Autodesk Fusion 360 part; units mm, degrees
note: some values were not read from the file. Set by a fixed rule: which face or edge a step refers to.
(part 2 of 5)
sketch "Sketch11" plane through (-60, 0, 0) normal (-1, 0, 0) x (0, 0, 1)
  line L0 (-42, 0) -> (42, 0)
  line L1 (42, 31) -> (-42, 31)
  line L2 (-42, 7) -> (-42, 10)
  line L3 (-42, 8.5) -> (41.5, 8.5) construction
  circle A0 centre (-29.5, 8.5) radius 1.5
  circle A1 centre (-24.5, 8.5) radius 1.5
  circle A2 centre (-19.5, 8.5) radius 1.5
  circle A3 centre (-14.5, 8.5) radius 1.5
  circle A4 centre (29.5, 8.5) radius 1.5
  circle A5 centre (24.5, 8.5) radius 1.5
  circle A6 centre (19.5, 8.5) radius 1.5
  circle A7 centre (14.5, 8.5) radius 1.5
  circle A8 centre (-29.5, 13.5) radius 1.5
  circle A9 centre (-24.5, 13.5) radius 1.5
  circle A10 centre (-19.5, 13.5) radius 1.5
  circle A11 centre (-14.5, 13.5) radius 1.5
  circle A12 centre (-29.5, 18.5) radius 1.5
  circle A13 centre (-24.5, 18.5) radius 1.5
  circle A14 centre (-19.5, 18.5) radius 1.5
  circle A15 centre (-14.5, 18.5) radius 1.5
  circle A16 centre (29.5, 13.5) radius 1.5
  circle A17 centre (24.5, 13.5) radius 1.5
  circle A18 centre (19.5, 13.5) radius 1.5
  circle A19 centre (14.5, 13.5) radius 1.5
  circle A20 centre (29.5, 18.5) radius 1.5
  circle A21 centre (24.5, 18.5) radius 1.5
  circle A22 centre (19.5, 18.5) radius 1.5
  circle A23 centre (14.5, 18.5) radius 1.5
  line L4 (-6, 5) -> (-6, 16)
  line L5 (-6, 16) -> (10, 16)
  line L6 (10, 16) -> (10, 5)
  line L7 (10, 5) -> (-6, 5)
  line L8 (42, 0) -> (42, 31)
  line L9 (-42, 31) -> (-42, 0)
  dimension "d84" = 3
  dimension "d87" = 15
  dimension "d88" = 10
  dimension "d91" = -15
  dimension "d92" = 10
  constraint midpoint L2 L3.start
  constraint coincident L3 A0.centre
  constraint coincident L3 A4.centre
  constraint equal A0 A4
  measures "d84" diameter of A0
extrude "Extrude10" cut sketch "Sketch11" against normal up to surface (8 mm away) contours A0 | A1 | A2 | A3 | A4 | A5 | A6 | A7 | A8 | A9 | A10 | A11 | A12 | A13 | A14 | A15 | A16 | A17 | A18 | A19 | A20 | A21 | A22 | A23 bodies 1
fillet "Fillet1" [suppressed]
fillet "Fillet2" [suppressed]
equation "d3 = d1 / 2"
equation "d4 = d2 / 2"
equation "d8 = d7"
equation "d9 = d7"
equation "d10 = d7"
equation "d18 = d17"
equation "d19 = d17"
equation "d20 = d17"
equation "d21 = d17 + 4 mm"
equation "d22 = d21"
equation "d23 = d21"
equation "d24 = d21"
equation "d25 = 8.00 mm"
equation "d27 = d25 - 1 mm"
equation "d32 = 2 mm"
equation "d33 = d32"
equation "d34 = d25"
equation "d40 = d39"
equation "d41 = d39"
equation "d42 = d39"
equation "d62 = d60 / 2"
equation "d63 = d61 / 2"
equation "d66 = d64"
equation "d68 = d67"
equation "d69 = d67"
equation "d70 = d67"

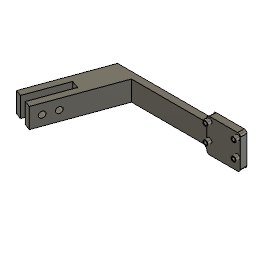
design "Camera Arm"
Autodesk Fusion 360 part; units mm, degrees
sketch "Sketch1" plane through (0, 0, 0) normal (0, 0, 1) x (1, 0, 0)
  circle A0 centre (10.5, -3.138) radius 1.2
  line L0 (-10.5, 12.5) -> (10.5, 12.5)
  arc A1 (-12.5, -10.5) -> (-10.5, -12.5) centre (-10.5, -10.5) ccw
  circle A2 centre (-10.5, -3.138) radius 1.2
  arc A3 (10.5, -12.5) -> (12.5, -10.5) centre (10.5, -10.5) ccw
  circle A4 centre (-10.5, 9.362) radius 1.2
  arc A5 (-10.5, 12.5) -> (-12.5, 10.5) centre (-10.5, 10.5) ccw
  line L1 (-12.5, -10.5) -> (-12.5, 10.5)
  line L2 (12.5, 10.5) -> (12.5, -10.5)
  arc A6 (12.5, 10.5) -> (10.5, 12.5) centre (10.5, 10.5) ccw
  circle A7 centre (10.5, 9.362) radius 1.2
  line L3 (10.5, -12.5) -> (-10.5, -12.5)
  point P0 (-12.5, 12.5)
  point P1 (12.5, 12.5)
  point P2 (-12.5, -12.5)
  dimension "d1" = 25
  dimension "d2" = 25
  dimension "d3" = 2.4
  dimension "d4" = 2
  dimension "d5" = 2
  dimension "d6" = 2
  dimension "d7" = 2
  dimension "d8" = 2
  dimension "d9" = 2
  dimension "d10" = 2
  dimension "d11" = 12.5
  dimension "d12" = 12.5
  dimension "d13" = 21.862
  dimension "d14" = 21.862
  dimension "d15" = 9.362
  dimension "d16" = 9.362
  dimension "d17" = 12.5
  dimension "d18" = 12.5
  constraint horizontal L0
  constraint vertical L2
  constraint horizontal L3
  constraint vertical L1
  constraint equal A2 A4
  constraint equal A0 A2
  constraint equal A0 A7
  constraint coincident P0 L0
  constraint coincident P0 L1
  constraint tangent L0 A5
  constraint tangent A5 L1
  constraint coincident P1 L0
  constraint coincident P1 L2
  constraint tangent L0 A6
  constraint tangent L2 A6
  constraint equal A5 A6
  constraint coincident P2 L3
  constraint coincident P2 L1
  constraint tangent A1 L3
  constraint tangent A1 L1
  constraint tangent A3 L2
  constraint tangent A3 L3
  measures "d1" distance of P0 P1
  measures "d2" distance of P0 P2
  measures "d3" diameter of A4
  measures "d4" distance of A7.centre L2
  measures "d5" distance of A0.centre L2
  measures "d6" distance of A2.centre L1
  measures "d7" distance of A4.centre L1
  measures "d8" radius of A5
  measures "d9" radius of A1
  measures "d10" radius of A3
  measures "d11" distance of origin L1
  measures "d12" distance of origin L0
  measures "d13" distance of A7.centre L3
  measures "d14" distance of A4.centre L3
  measures "d15" distance of A0.centre L3
  measures "d16" distance of A2.centre L3
  measures "d17" distance of origin L1
  measures "d18" distance of origin L0
extrude "Extrude1" add sketch "Sketch1" along normal blind 5
sketch "Sketch2" plane through (0, 0, 5) normal (0, 0, 1) x (1, 0, 0)
  circle A0 centre (-10.5, 9.362) radius 1.2
  circle A1 centre (10.5, -3.138) radius 1.2
  circle A2 centre (-10.5, -3.138) radius 1.2
  circle A3 centre (10.5, 9.362) radius 1.2
  arc A4 (12.5, 10.5) -> (10.5, 12.5) centre (10.5, 10.5) ccw
  line L0 (10.5, 12.5) -> (-10.5, 12.5)
  arc A5 (-10.5, 12.5) -> (-12.5, 10.5) centre (-10.5, 10.5) ccw
  line L1 (-12.5, 10.5) -> (-12.5, -10.5)
  arc A6 (-12.5, -10.5) -> (-10.5, -12.5) centre (-10.5, -10.5) ccw
  line L2 (-10.5, -12.5) -> (10.5, -12.5)
  arc A7 (10.5, -12.5) -> (12.5, -10.5) centre (10.5, -10.5) ccw
  line L3 (12.5, -10.5) -> (12.5, 10.5)
  circle A8 centre (-10.5, 9.362) radius 1.85
  circle A9 centre (10.5, 9.362) radius 1.85
  circle A10 centre (10.5, -3.138) radius 1.85
  circle A11 centre (-10.5, -3.138) radius 1.85
  dimension "d21" = 3.7
  dimension "d22" = 3.7
  dimension "d23" = 3.7
  dimension "d24" = 3.7
  constraint concentric A0 A8
  constraint concentric A3 A9
  constraint concentric A1 A10
  constraint concentric A2 A11
  measures "d21" diameter of A8
  measures "d22" diameter of A9
  measures "d23" diameter of A10
  measures "d24" diameter of A11
extrude "Extrude2" add sketch "Sketch2" along normal blind 3 contours A8 | A9 | A10 | A11
sketch "Sketch3" plane through (-12.5, 0, 0) normal (-1, 0, 0) x (0, 0, 1)
  line L0 (0, 10.5) -> (0, -10.5)
  line L1 (0, -10.5) -> (5, -10.5)
  line L2 (5, -10.5) -> (5, 10.5)
  line L3 (5, 10.5) -> (0, 10.5)
  line L4 (0, 7.5) -> (5, 7.5)
  line L5 (5, 7.5) -> (5, -7.5)
  line L6 (5, -7.5) -> (0, -7.5)
  line L7 (0, -7.5) -> (0, 7.5)
  dimension "d29" = 3
  dimension "d30" = 3
  constraint horizontal L4
  constraint vertical L5
  constraint horizontal L6
  constraint vertical L7
  constraint coincident L2 L5.end
  constraint coincident L0 L4.start
  measures "d29" distance of L3 L4
  measures "d30" distance of L1 L6
extrude "Extrude3" add sketch "Sketch3" along normal blind 68 contours L0 L2 L4 L5 L6 L7
fillet "Fillet1" radius 3 2 edges at (-12.5, 7.5, 2.5) (-12.5, -7.5, 2.5)
sketch "Sketch5" plane through (0, 7.5, 0) normal (0, 1, 0) x (-1, 0, 0)
  line L0 (15.5, 5) -> (15.5, 0)
  line L1 (15.5, 0) -> (80.5, 0)
  line L2 (80.5, 0) -> (80.5, 5)
  line L3 (80.5, 5) -> (15.5, 5)
  line L4 (80.5, 0) -> (94.2374, 0)
  line L5 (94.2374, 0) -> (80.5, 5)
  line L6 (84.001, 0) -> (85.1985, 3.2899)
  dimension "d38" = 20
  dimension "d39" = 5
  dimension "d40" = 5
  constraint coincident L1.end L2.start
  constraint perpendicular L2 L4
  constraint coincident L2.end L3.start
  constraint coincident L4 L6.start
  constraint coincident L5 L6.end
  constraint perpendicular L5 L6
  measures "d38" angle of L4 L5
  measures "d39" distance of L1.end L2.end
  measures "d40" distance of L2.end L6.end
extrude "Extrude5" add sketch "Sketch5" against normal up to surface (15 mm away) contours L2 L4 L5 L6
sketch "Sketch6" plane through (-11.0237, 0, 30.2873) normal (-0.34202, 0, 0.939693) x (0.939693, 0, 0.34202)
  line L0 (-78.9352, -7.5) -> (-73.9352, -7.5)
  line L1 (-73.9352, -7.5) -> (-73.9352, 7.5)
  line L2 (-73.9352, 7.5) -> (-78.9352, 7.5)
  line L3 (-78.9352, 7.5) -> (-78.9352, -7.5)
  line L4 (-78.9352, 7.5) -> (-73.9352, 7.5)
  line L5 (-73.9352, 7.5) -> (-73.9352, -7.5)
  line L6 (-73.9352, -7.5) -> (-78.9352, -7.5)
  line L7 (-78.9352, -7.5) -> (-78.9352, 7.5)
  constraint horizontal L4
  constraint vertical L5
  constraint horizontal L6
  constraint vertical L7
  constraint coincident L0.end L1.start
  constraint coincident L2.end L3.start
extrude "Extrude6" add sketch "Sketch6" along normal blind 55.398
sketch "Sketch7" plane through (-69.4763, 0, -25.2873) normal (0.939693, 0, 0.34202) x (0.34202, 0, -0.939693)
  line L0 (-32.2311, -7.5) -> (-32.2311, 7.5)
  line L1 (-32.2311, 7.5) -> (-87.6291, 7.5)
  line L2 (-87.6291, 7.5) -> (-87.6291, -7.5)
  line L3 (-87.6291, -7.5) -> (-32.2311, -7.5)
  line L4 (-87.6291, 0) -> (-32.2311, 0) construction
  circle A0 centre (-80.1291, 0) radius 2.25
  circle A1 centre (-70.1291, 0) radius 2.25
  dimension "d45" = 4.5
  dimension "d46" = 4.5
  dimension "d47" = 7.5
  dimension "d48" = 10
  constraint midpoint L2 L4.start
  constraint midpoint L0 L4.end
  constraint coincident L4 A0.centre
  constraint coincident L4 A1.centre
  measures "d45" diameter of A0
  measures "d46" diameter of A1
  measures "d47" distance of L2 A0.centre
  measures "d48" distance of A0.centre A1.centre
extrude "Extrude7" cut sketch "Sketch7" against normal up to surface (5 mm away) contours A0 | A1
sketch "Sketch8" plane through (0, 7.5, 0) normal (0, 1, 0) x (-1, 0, 0)
  line L0 (15.5, 5) -> (15.5, 0)
  line L1 (15.5, 0) -> (84.001, 0)
  line L2 (84.001, 0) -> (104.1457, 55.347)
  line L3 (104.1457, 55.347) -> (99.4472, 57.0571)
  line L4 (99.4472, 57.0571) -> (80.5, 5)
  line L5 (80.5, 5) -> (15.5, 5)
  line L6 (74.0085, 5) -> (93.7151, 59.1434)
  line L7 (93.7151, 59.1434) -> (89.0166, 60.8535)
  line L8 (89.0166, 60.8535) -> (68.6876, 5)
  line L9 (99.4472, 57.0571) -> (93.7151, 59.1434) construction
  dimension "d51" = 6.1
  dimension "d52" = 5
  constraint coincident L5 L6.start
  constraint perpendicular L6 L7
  constraint coincident L5 L8.end
  constraint parallel L4 L6
  constraint perpendicular L7 L8
  constraint coincident L3.end L4.start
  constraint perpendicular L4 L9
  measures "d51" distance of L4 L6
  measures "d52" distance of L6.end L7.end
extrude "Extrude8" add sketch "Sketch8" against normal up to surface (15 mm away) contours L5 L6 L7 L8
sketch "Sketch9" plane through (-59.0457, 0, -21.4909) normal (0.939693, 0, 0.34202) x (0.34202, 0, -0.939693)
  line L0 (-87.6291, -7.5) -> (-28.191, -7.5)
  line L1 (-28.191, -7.5) -> (-28.191, 7.5)
  line L2 (-28.191, 7.5) -> (-87.6291, 7.5)
  line L3 (-87.6291, 7.5) -> (-87.6291, -7.5)
  circle A0 centre (-80.1291, 0) radius 2.25
  circle A1 centre (-70.1291, 0) radius 2.25
extrude "Extrude9" cut sketch "Sketch9" against normal up to surface (5 mm away) contours A0 | A1
sketch "Sketch10" plane through (0, 7.5, 0) normal (0, 1, 0) x (-1, 0, 0)
  line L0 (15.5, 5) -> (15.5, 0)
  line L1 (15.5, 0) -> (84.001, 0)
  line L2 (84.001, 0) -> (104.1457, 55.347)
  line L3 (104.1457, 55.347) -> (99.4472, 57.0571)
  line L4 (99.4472, 57.0571) -> (80.5, 5)
  line L5 (80.5, 5) -> (74.0085, 5)
  line L6 (74.0085, 5) -> (93.7151, 59.1434)
  line L7 (93.7151, 59.1434) -> (89.0166, 60.8535)
  line L8 (89.0166, 60.8535) -> (68.6876, 5)
  line L9 (68.6876, 5) -> (15.5, 5)
  line L10 (89.0505, 28.4923) -> (83.3184, 30.5786)
  dimension "d57" = 30.398
  constraint coincident L4 L10.start
  constraint coincident L6 L10.end
  constraint perpendicular L6 L10
  measures "d57" distance of L3 L10
extrude "Extrude10" add sketch "Sketch10" against normal up to surface (15 mm away) contours L4 L5 L6 L10
equation "d17 = d11"
equation "d18 = d12"
equation "d22 = d21"
equation "d23 = d21"
equation "d24 = d21"
equation "d30 = d29"
equation "d40 = d39"
equation "d43 = 19.898 mm + 7.5 mm + 28 mm"
equation "d46 = d45"
equation "d57 = d43 - 25 mm"

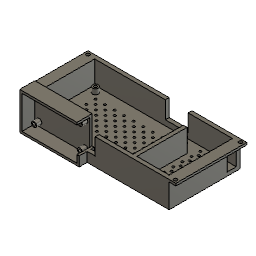
design "PCB Case"
Autodesk Fusion 360 part; units mm, degrees
sketch "Sketch1" plane through (0, 0, 0) normal (0, 1, 0) x (1, 0, 0)
  line L0 (-72.5, 44.98) -> (120.5, 44.98)
  line L1 (120.5, 44.98) -> (120.5, -49.32)
  line L2 (120.5, -49.32) -> (-72.5, -49.32)
  line L3 (-72.5, -49.32) -> (-72.5, 44.98)
  line L4 (-67.5, 39.83) -> (67.5, 39.83)
  line L5 (67.5, 39.83) -> (67.5, -39.83)
  line L6 (67.5, -39.83) -> (-67.5, -39.83)
  line L7 (-67.5, -39.83) -> (-67.5, 39.83)
  circle A0 centre (-58.42, 31.75) radius 1.9
  circle A1 centre (-58.42, -31.75) radius 1.9
  circle A2 centre (58.42, 31.75) radius 1.9
  circle A3 centre (58.42, -31.75) radius 1.9
  circle A4 centre (-58.42, 31.75) radius 3.9
  circle A5 centre (58.42, 31.75) radius 3.9
  circle A6 centre (58.42, -31.75) radius 3.9
  circle A7 centre (-58.42, -31.75) radius 3.9
  line L8 (72.5, 39.83) -> (115.5, 39.83)
  line L9 (115.5, 39.83) -> (115.5, -44.17)
  line L10 (115.5, -44.17) -> (72.5, -44.17)
  line L11 (72.5, -44.17) -> (72.5, 39.83)
  line L12 (67.5, 39.83) -> (72.5, 39.83) construction
  dimension "d1" = 135
  dimension "d2" = 67.5
  dimension "d3" = 79.66
  dimension "d4" = 39.83
  dimension "d5" = 5.15
  dimension "d8" = 5
  dimension "d9" = 58.42
  dimension "d10" = 58.42
  dimension "d11" = 58.42
  dimension "d12" = 58.42
  dimension "d13" = 31.75
  dimension "d14" = 31.75
  dimension "d15" = 31.75
  dimension "d16" = 31.75
  dimension "d17" = 3.8
  dimension "d18" = 3.8
  dimension "d19" = 3.8
  dimension "d20" = 3.8
  dimension "d21" = 7.8
  dimension "d22" = 7.8
  dimension "d23" = 7.8
  dimension "d24" = 7.8
  dimension "d111" = 43
  dimension "d112" = 84
  dimension "d113" = 5.15
  dimension "d114" = 5
  dimension "d115" = 5
  constraint horizontal L0
  constraint vertical L1
  constraint horizontal L2
  constraint vertical L3
  constraint horizontal L4
  constraint vertical L5
  constraint horizontal L6
  constraint vertical L7
  constraint concentric A0 A4
  constraint concentric A2 A5
  constraint concentric A3 A6
  constraint concentric A1 A7
  constraint horizontal L8
  constraint vertical L9
  constraint horizontal L10
  constraint vertical L11
  constraint horizontal L12
  measures "d1" distance of L4.start L4.end
  measures "d2" distance of origin L5
  measures "d3" distance of L4.start L6.end
  measures "d4" distance of origin L4
  measures "d5" distance of L0 L4
  measures "d8" distance of L3 L7
  measures "d9" horizontal distance of origin A0.centre
  measures "d10" horizontal distance of origin A2.centre
  measures "d11" horizontal distance of origin A1.centre
  measures "d12" horizontal distance of origin A3.centre
  measures "d13" vertical distance of origin A0.centre
  measures "d14" vertical distance of origin A2.centre
  measures "d15" vertical distance of origin A1.centre
  measures "d16" vertical distance of origin A3.centre
  measures "d17" diameter of A0
  measures "d18" diameter of A2
  measures "d19" diameter of A1
  measures "d20" diameter of A3
  measures "d21" diameter of A4
  measures "d22" diameter of A5
  measures "d23" diameter of A7
  measures "d24" diameter of A6
  measures "d111" distance of L8.start L8.end
  measures "d112" distance of L8.end L9.end
  measures "d113" distance of L2 L10
  measures "d114" distance of L1 L9
  measures "d115" distance of L5 L11
extrude "Extrude1" add sketch "Sketch1" along normal blind 5 contours L4 L5 L6 L7 | A4 | A5 | A6 | A7 | L8 L9 L10 L11 makes body 1 at (-18.887, 0, 10.2448) makes body 2 at (86.8333, 0, 16.17)
extrude "Extrude3" add sketch "Sketch1" along normal blind 35 contours L0 L1 L2 L3 bodies 1 2
extrude "Extrude15" add sketch "Sketch1" along normal blind 5 contours A0 | A1 | A2 | A3 bodies 1
extrude "Extrude16" add sketch "Sketch1" along normal blind 12 contours A4 | A5 | A6 | A7 bodies 1
sketch "Sketch11" plane through (0, 35, 0) normal (0, 1, 0) x (-1, 0, 0)
  line L0 (-67.5, 39.83) -> (67.5, 39.83)
  line L1 (67.5, 39.83) -> (67.5, -39.83)
  line L2 (67.5, -39.83) -> (-67.5, -39.83)
  line L3 (-67.5, -39.83) -> (-67.5, 39.83)
  line L4 (-115.5, 44.17) -> (-72.5, 44.17)
  line L5 (-72.5, 44.17) -> (-72.5, -39.83)
  line L6 (-72.5, -39.83) -> (-115.5, -39.83)
  line L7 (-115.5, -39.83) -> (-115.5, 44.17)
  line L8 (72.5, 49.32) -> (-120.5, 49.32)
  line L9 (-120.5, 49.32) -> (-120.5, -44.98)
  line L10 (-120.5, -44.98) -> (72.5, -44.98)
  line L11 (72.5, -44.98) -> (72.5, 49.32)
  line L12 (72.5, 49.32) -> (-67.5, 49.32)
  line L13 (-67.5, 49.32) -> (-67.5, 44.83)
  line L14 (-67.5, 44.83) -> (72.5, 44.83)
  line L15 (72.5, 44.83) -> (72.5, 49.32)
  line L16 (-67.5, 44.83) -> (-67.5, 39.83)
  dimension "d117" = 5
  constraint horizontal L12
  constraint vertical L13
  constraint horizontal L14
  constraint vertical L15
  constraint coincident L8.start L11.end
  constraint coincident L0.start L3.end
  constraint vertical L16
  measures "d117" distance of L0 L14
extrude "Extrude11" cut sketch "Sketch11" against normal up to surface (35 mm away) contours L8 L11 L12 L13 L14 L15 bodies 1
sketch "Sketch2" plane through (0, 35, 0) normal (0, 1, 0) x (-1, 0, 0)
  line L0 (-67.5, 39.83) -> (67.5, 39.83)
  line L1 (67.5, 39.83) -> (67.5, -39.83)
  line L2 (67.5, -39.83) -> (-67.5, -39.83)
  line L3 (-67.5, -39.83) -> (-67.5, 39.83)
  line L4 (-67.5, 49.32) -> (-120.5, 49.32)
  line L5 (-120.5, 49.32) -> (-120.5, -44.98)
  line L6 (-120.5, -44.98) -> (72.5, -44.98)
  line L7 (72.5, -44.98) -> (72.5, 44.83)
  line L8 (81.5, -44.98) -> (-129.5, -44.98)
  line L9 (-129.5, -44.98) -> (-129.5, 49.32)
  line L10 (81.5, 44.83) -> (81.5, -44.98)
  circle A0 centre (77, 40.33) radius 2.25
  circle A1 centre (77, -40.48) radius 2.25
  circle A2 centre (-125, -40.98) radius 2.25
  circle A3 centre (-125, 45.32) radius 2.25
  line L11 (-115.5, 44.17) -> (-72.5, 44.17)
  line L12 (-72.5, 44.17) -> (-72.5, -39.83)
  line L13 (-72.5, -39.83) -> (-115.5, -39.83)
  line L14 (-115.5, -39.83) -> (-115.5, 44.17)
  line L15 (-67.5, 44.83) -> (-67.5, 49.32)
  line L16 (72.5, 44.83) -> (-67.5, 44.83)
  line L17 (-129.5, 49.32) -> (-120.5, 49.32)
  line L18 (72.5, 44.83) -> (81.5, 44.83)
  point P0 (-24, -44.98)
  dimension "d33" = 9
  dimension "d39" = 4.5
  dimension "d40" = 4.5
  dimension "d41" = 4.5
  dimension "d42" = 4.5
  dimension "d43" = 4
  dimension "d44" = 4.5
  dimension "d46" = 4.5
  dimension "d47" = 4.5
  dimension "d48" = 4.5
  dimension "d50" = 4.5
  dimension "d116" = 9
  dimension "d121" = 4
  dimension "d122" = 4.5
  constraint horizontal L8
  constraint vertical L9
  constraint vertical L10
  constraint midpoint L6 P0
  constraint coincident L8 P0
  constraint coincident L4.end L5.start
  constraint perpendicular L5 L17
  constraint coincident L7.end L16.start
  constraint horizontal L18
  measures "d33" distance of L7 L10
  measures "d39" distance of L10 A1.centre
  measures "d40" distance of L8 A1.centre
  measures "d41" diameter of A1
  measures "d42" distance of L9 A2.centre
  measures "d43" distance of L8 A2.centre
  measures "d44" diameter of A2
  measures "d46" distance of L10 A0.centre
  measures "d47" diameter of A0
  measures "d48" distance of L9 A3.centre
  measures "d50" diameter of A3
  measures "d116" distance of L5 L9
  measures "d121" distance of A3.centre L17
  measures "d122" distance of A0.centre L18
extrude "Extrude4" add sketch "Sketch2" against normal blind 3 contours L5 L8 L9 L17 | L7 L8 L10 L18 bodies 1
sketch "Sketch7" plane through (0, 35, 0) normal (0, 1, 0) x (-1, 0, 0)
  line L0 (81.5, -44.98) -> (81.5, 44.83)
  line L1 (-67.5, 49.32) -> (-129.5, 49.32)
  circle A0 centre (77, 40.33) radius 2.25
  line L2 (67.5, 39.83) -> (-11.62, 39.83)
  line L3 (67.5, 59.83) -> (67.5, 39.83)
  line L4 (-11.62, 39.83) -> (-11.62, 59.83)
  line L5 (67.5, 59.83) -> (-11.62, 59.83)
  line L6 (-129.5, -44.98) -> (81.5, -44.98)
  circle A1 centre (77, -40.48) radius 2.25
  line L7 (-67.5, -39.83) -> (-67.5, 39.83)
  line L8 (-67.5, 39.83) -> (67.5, 39.83)
  line L9 (67.5, 39.83) -> (67.5, -39.83)
  line L10 (67.5, -39.83) -> (-67.5, -39.83)
  line L11 (81.5, 44.83) -> (-67.5, 44.83)
  line L12 (-67.5, 44.83) -> (-67.5, 49.32)
  line L13 (-129.5, 49.32) -> (-129.5, -44.98)
  circle A2 centre (-125, 45.32) radius 2.25
  circle A3 centre (-125, -40.98) radius 2.25
  line L14 (-115.5, 44.17) -> (-72.5, 44.17)
  line L15 (-72.5, 44.17) -> (-72.5, -39.83)
  line L16 (-72.5, -39.83) -> (-115.5, -39.83)
  line L17 (-115.5, -39.83) -> (-115.5, 44.17)
  dimension "d59" = 20
  dimension "d60" = 79.12
  constraint horizontal L2
  constraint vertical L3
  constraint perpendicular L3 L5
  constraint coincident L2 L3.end
  constraint coincident L3 L2.start
  constraint perpendicular L4 L5
  measures "d59" distance of L2.start L3.start
  measures "d60" distance of L2.start L2.end
extrude "Extrude6" add sketch "Sketch7" against normal up to surface (35 mm away) contours L3 L4 L5 L11 bodies 1
extrude "Extrude7" add sketch "Sketch7" along normal blind 14.91 contours L3 L4 L5 L11 | L2 L3 L4 L8 L11 bodies 1
sketch "Sketch8" plane through (0, 0, 59.83) normal (0, 0, 1) x (1, 0, 0)
  line L0 (11.62, 0) -> (11.62, 49.91)
  line L1 (11.62, 49.91) -> (-67.5, 49.91)
  line L2 (-67.5, 49.91) -> (-67.5, 0)
  line L3 (-64.5, 46.91) -> (8.62, 46.91)
  line L4 (8.62, 46.91) -> (8.62, 3)
  line L5 (8.62, 3) -> (-64.5, 3)
  line L6 (-64.5, 3) -> (-64.5, 46.91)
  line L7 (-67.5, 0) -> (11.62, 0)
  dimension "d65" = 3
  dimension "d66" = 3
  dimension "d67" = 3
  dimension "d140" = 3
  constraint horizontal L3
  constraint vertical L4
  constraint horizontal L5
  constraint vertical L6
  measures "d65" distance of L2 L6
  measures "d66" distance of L1 L3
  measures "d67" distance of L0 L4
  measures "d140" distance of L5 L7
extrude "Extrude8" cut sketch "Sketch8" against normal blind 17 contours L3 L4 L5 L6 bodies 1
sketch "Sketch9" plane through (0, 0, 42.83) normal (0, 0, 1) x (1, 0, 0)
  line L0 (-64.5, 3) -> (8.62, 3)
  line L1 (8.62, 3) -> (8.62, 46.91)
  line L2 (-64.5, 46.91) -> (-64.5, 3)
  circle A0 centre (-58.42, 40.83) radius 1.9
  circle A1 centre (2.54, 40.83) radius 1.9
  circle A2 centre (-58.42, 9.08) radius 1.9
  circle A3 centre (2.54, 9.08) radius 1.9
  line L3 (-64.5, 24.955) -> (8.62, 24.955) construction
  line L4 (8.62, 46.91) -> (-64.5, 46.91)
  circle A4 centre (-58.42, 9.08) radius 3.4
  circle A5 centre (-58.42, 40.83) radius 3.4
  circle A6 centre (2.54, 40.83) radius 3.4
  circle A7 centre (2.54, 9.08) radius 3.4
  line L5 (-13.97, 31.94) -> (-62.23, 31.94)
  line L6 (-62.23, 31.94) -> (-62.23, 37.02)
  line L7 (-62.23, 37.02) -> (-26.67, 37.02)
  line L8 (-26.67, 37.02) -> (-26.67, 43.37)
  line L9 (-26.67, 43.37) -> (-13.97, 43.37)
  line L10 (-13.97, 43.37) -> (-13.97, 31.94)
  dimension "d79" = 3.8
  dimension "d80" = 3.8
  dimension "d81" = 3.8
  dimension "d82" = 3.8
  dimension "d85" = 6.08
  dimension "d86" = 6.08
  dimension "d87" = 6.08
  dimension "d88" = 6.08
  dimension "d89" = 6.08
  dimension "d91" = 6.08
  dimension "d131" = 6.08
  dimension "d132" = 6.08
  dimension "d133" = 6.8
  dimension "d134" = 6.8
  dimension "d135" = 6.8
  dimension "d136" = 6.8
  dimension "d138" = 22.86
  dimension "d141" = 5.08
  dimension "d142" = 3.81
  dimension "d143" = 31.75
  dimension "d144" = 12.7
  dimension "d145" = 2.54
  constraint midpoint L2 L3.start
  constraint midpoint L1 L3.end
  constraint concentric A2 A4
  constraint concentric A0 A5
  constraint concentric A1 A6
  constraint concentric A3 A7
  constraint horizontal L5
  constraint vertical L6
  constraint perpendicular L6 L7
  constraint perpendicular L7 L8
  constraint perpendicular L8 L9
  constraint perpendicular L9 L10
  measures "d79" diameter of A2
  measures "d80" diameter of A0
  measures "d81" diameter of A1
  measures "d82" diameter of A3
  measures "d85" distance of L0 A2.centre
  measures "d86" distance of L2 A2.centre
  measures "d87" distance of L0 A3.centre
  measures "d88" distance of L1 A3.centre
  measures "d89" distance of L2 A0.centre
  measures "d91" distance of L1 A1.centre
  measures "d131" distance of A0.centre L4
  measures "d132" distance of A1.centre L4
  measures "d133" diameter of A4
  measures "d134" diameter of A5
  measures "d135" diameter of A6
  measures "d136" diameter of A7
  measures "d138" distance of A2.centre L5
  measures "d141" distance of L6.end L5.end
  measures "d142" distance of A0.centre L6
  measures "d143" distance of A0.centre L8
  measures "d144" distance of L8.end L9.end
  measures "d145" distance of A0.centre L9
extrude "Extrude9" add sketch "Sketch9" along normal blind 7 contours A4 | A5 | A6 | A7 bodies 1
extrude "Extrude14" cut sketch "Sketch9" against normal up to surface (3 mm away) contours L5 L6 L7 L8 L9 L10 bodies 1
sketch "Sketch5" plane through (0, 0, -44.98) normal (0, 0, -1) x (-1, 0, 0)
  line L0 (72.5, 32) -> (81.5, 32)
  line L1 (-120.5, 32) -> (-120.5, 0)
  line L2 (-120.5, 0) -> (72.5, 0)
  line L3 (72.5, 0) -> (72.5, 32)
  line L4 (81.5, 35) -> (-129.5, 35)
  line L5 (72.5, 32) -> (81.5, 32)
  line L6 (81.5, 32) -> (81.5, 35)
  line L7 (81.5, 32) -> (81.5, 35)
  line L8 (81.5, 35) -> (-129.5, 35)
  line L9 (-120.5, 0) -> (72.5, 0)
  line L10 (72.5, 0) -> (72.5, 32)
  line L11 (-120.5, 32) -> (-120.5, 0)
  line L12 (-56.52, 12) -> (-26.52, 12)
  line L13 (-26.52, 12) -> (-26.52, 35)
  line L14 (-26.52, 35) -> (-56.52, 35)
  line L15 (-56.52, 35) -> (-56.52, 12)
  line L16 (-56.52, 5) -> (-56.52, 35) construction
  line L17 (-129.5, 35) -> (-129.5, 32)
  line L18 (-129.5, 32) -> (-120.5, 32)
  line L19 (-129.5, 35) -> (-129.5, 32)
  line L20 (-129.5, 32) -> (-120.5, 32)
  line L21 (-72.5, 5) -> (-115.5, 5)
  line L22 (-115.5, 5) -> (-72.5, 5)
  line L23 (-60.32, 12) -> (-56.52, 12)
  line L24 (-54.52, 12) -> (-62.32, 12)
  dimension "d95" = 30
  constraint horizontal L12
  constraint vertical L13
  constraint horizontal L14
  constraint vertical L15
  constraint coincident L8 L13.end
  constraint coincident L4 L14.end
  constraint perpendicular L4 L16
  constraint coincident L12.start L16
  constraint coincident L12 L24.start
  constraint coincident L15 L12.start
  measures "d95" distance of L13.end L14.end
extrude "Extrude5" cut sketch "Sketch5" along normal up to surface (0 mm away) and the other way up to surface (5.15 mm away) contours L4 L8 L12 L13 L14 L15 L24 bodies 1
sketch "Sketch10" plane through (0, 0, 49.32) normal (0, 0, 1) x (1, 0, 0)
  line L0 (129.5, 35) -> (67.5, 35)
  line L1 (8.62, 3) -> (8.62, 46.91)
  line L2 (8.62, 46.91) -> (8.62, 3)
  line L3 (22.23, 49.91) -> (8.62, 49.91)
  line L4 (8.62, 49.91) -> (8.62, 12.874)
  line L5 (8.62, 12.874) -> (22.23, 12.874)
  line L6 (11.62, 49.91) -> (-67.5, 49.91)
  line L7 (11.62, 49.91) -> (24.4054, 49.91) construction
  line L8 (22.23, 49.91) -> (22.23, 12.874)
  line L9 (67.5, 0) -> (120.5, 0)
  line L10 (120.5, 0) -> (120.5, 32)
  line L11 (120.5, 32) -> (129.5, 32)
  line L12 (-67.5, 49.91) -> (11.62, 49.91)
  line L13 (67.5, 35) -> (67.5, 0)
  line L14 (129.5, 32) -> (129.5, 35)
  line L15 (72.5, 5) -> (115.5, 5)
  line L16 (115.5, 5) -> (72.5, 5)
  constraint horizontal L3
  constraint vertical L4
  constraint horizontal L5
  constraint coincident L2 L4.end
  constraint coincident L6.start L7.start
  constraint parallel L6 L7
  constraint coincident L3.start L7
  constraint perpendicular L3 L8
extrude "Extrude10" cut sketch "Sketch10" along normal up to surface (-9.49 mm away) and the other way up to surface (-10.51 mm away) contours L1 L2 L3 L4 L5 L6 L8 L12 bodies 1
sketch "Sketch12" plane through (120.5, 0, 0) normal (1, 0, 0) x (0, 0, -1)
  line L0 (44.98, 32) -> (-49.32, 32)
  line L1 (-44.17, 5) -> (39.83, 5)
  line L2 (39.83, 5) -> (-44.17, 5)
  line L3 (-49.32, 32) -> (44.98, 32)
  line L4 (43.23, 32) -> (38.73, 32)
  line L5 (-43.07, 32) -> (-47.57, 32)
  line L6 (39.83, 5) -> (27.83, 5)
  line L7 (27.83, 5) -> (27.83, 25)
  line L8 (27.83, 25) -> (39.83, 25)
  line L9 (39.83, 25) -> (39.83, 5)
  line L10 (-49.32, 32) -> (-49.32, 0)
  line L11 (-49.32, 0) -> (44.98, 0)
  line L12 (44.98, 0) -> (44.98, 32)
  line L13 (44.98, 32) -> (-49.32, 32)
  dimension "d123" = 12
  dimension "d158" = 20
  constraint horizontal L6
  constraint vertical L7
  constraint horizontal L8
  constraint vertical L9
  constraint coincident L1.end L2.start
  measures "d123" distance of L1.end L6.end
  measures "d158" distance of L1.end L8.end
extrude "Extrude12" cut sketch "Sketch12" against normal up to surface (5 mm away) contours L1 L2 L6 L7 L8 L9 bodies 1
sketch "Sketch14" plane through (0, 0, 0) normal (0, -1, 0) x (1, 0, 0)
  line L0 (67.5, 44.83) -> (11.62, 44.83)
  line L1 (11.62, 44.83) -> (11.62, 59.83)
  line L2 (11.62, 59.83) -> (-67.5, 59.83)
  line L3 (-67.5, 59.83) -> (-67.5, 44.83)
  line L4 (-67.5, 44.83) -> (-72.5, 44.83)
  line L5 (-72.5, 44.83) -> (-72.5, -44.98)
  line L6 (-72.5, -44.98) -> (120.5, -44.98)
  line L7 (120.5, -44.98) -> (120.5, 49.32)
  line L8 (120.5, 49.32) -> (67.5, 49.32)
  line L9 (67.5, 49.32) -> (67.5, 44.83)
  line L10 (11.62, 44.83) -> (67.5, 44.83)
  line L11 (67.5, 44.83) -> (67.5, 49.32)
  line L12 (67.5, 49.32) -> (11.62, 49.32)
  line L13 (11.62, 49.32) -> (11.62, 44.83)
  line L14 (22.23, 44.83) -> (22.23, 49.32)
  point P0 (22.23, 44.83)
  constraint horizontal L10
  constraint vertical L11
  constraint horizontal L12
  constraint vertical L13
  constraint coincident L8.end L9.start
  constraint coincident L0.end L1.start
  constraint coincident P0 L14.start
  constraint coincident L12 L14.end
  constraint perpendicular L12 L14
extrude "Extrude17" add sketch "Sketch14" against normal up to surface (35 mm away) contours L0 L9 L10 L11 L12 L14 bodies 1
extrude "Extrude19" add sketch "Sketch14" against normal up to surface (12.874 mm away) contours L0 L1 L10 L12 L13 L14 bodies 1
sketch "Sketch15" plane through (0, 35, 0) normal (0, 1, 0) x (-1, 0, 0)
  line L0 (-115.5, 44.17) -> (-72.5, 44.17)
  line L1 (-72.5, 44.17) -> (-72.5, -39.83)
  line L2 (-72.5, -39.83) -> (-115.5, -39.83)
  line L3 (-115.5, -39.83) -> (-115.5, 44.17)
  circle A0 centre (-125, -40.98) radius 2.25
  circle A1 centre (-125, 45.32) radius 2.25
  line L4 (-22.23, 39.83) -> (-22.23, 49.32)
  line L5 (-22.23, 49.32) -> (-129.5, 49.32)
  line L6 (-129.5, 49.32) -> (-129.5, -44.98)
  line L7 (-129.5, -44.98) -> (-56.52, -44.98)
  line L8 (-56.52, -44.98) -> (-56.52, -39.83)
  line L9 (-56.52, -39.83) -> (-67.5, -39.83)
  line L10 (-67.5, -39.83) -> (-67.5, 39.83)
  line L11 (-67.5, 39.83) -> (-22.23, 39.83)
  line L12 (-11.62, 44.17) -> (-67.5, 44.17)
  line L13 (-67.5, 44.17) -> (-67.5, 39.83)
  line L14 (-67.5, 39.83) -> (-11.62, 39.83)
  line L15 (-11.62, 39.83) -> (-11.62, 44.17)
  line L16 (-72.5, 44.17) -> (-67.5, 44.17)
  line L17 (-22.23, 49.32) -> (-22.23, 39.83) construction
  line L18 (-22.23, 39.83) -> (-8.62, 39.83) construction
  line L19 (-8.62, 39.83) -> (-8.62, 42.83) construction
  line L20 (-8.62, 42.83) -> (-8.62, 59.83) construction
  line L21 (-8.62, 59.83) -> (-11.62, 59.83) construction
  line L22 (-11.62, 59.83) -> (-11.62, 49.32) construction
  line L23 (-11.62, 49.32) -> (-22.23, 49.32) construction
  line L24 (-11.62, 44.17) -> (-11.62, 49.32) construction
  constraint horizontal L12
  constraint vertical L13
  constraint horizontal L14
  constraint vertical L15
  constraint coincident L10.end L11.start
  constraint coincident L0.end L1.start
  constraint horizontal L16
  constraint coincident L22.end L23.start
  constraint vertical L24
extrude "Extrude18" cut sketch "Sketch15" against normal up to surface (30 mm away) contours L4 L11 L12 L13 L14 | L4 L12 L14 L15 bodies 1
sketch "Sketch16" plane through (67.5, 0, 0) normal (-1, 0, 0) x (0, 0, 1)
  line L0 (-39.83, 5) -> (44.17, 5)
  line L1 (44.17, 5) -> (44.17, 35)
  line L2 (44.17, 35) -> (-39.83, 35)
  line L3 (-39.83, 35) -> (-39.83, 5)
  line L4 (-39.83, 35) -> (-22.83, 35)
  line L5 (-22.83, 35) -> (-22.83, 5)
  line L6 (-22.83, 5) -> (-39.83, 5)
  line L7 (-39.83, 5) -> (-39.83, 35)
  line L8 (-39.83, 25) -> (-27.83, 25)
  dimension "d188" = 5
  constraint horizontal L4
  constraint vertical L5
  constraint horizontal L6
  constraint vertical L7
  constraint coincident L0 L5.end
  constraint coincident L2.end L3.start
  measures "d188" distance of L5 L8.end
extrude "Extrude20" cut sketch "Sketch16" against normal up to surface (5 mm away) contours L0 L2 L3 L4 L5 L6 L7 bodies 1
sketch "Sketch17" plane through (0, 5, 0) normal (0, 1, 0) x (-1, 0, 0)
  circle A0 centre (58.42, -31.75) radius 3.9
  circle A1 centre (58.42, 31.75) radius 3.9
  line L0 (67.5, 39.83) -> (-11.62, 39.83)
  line L1 (-11.62, 39.83) -> (-11.62, 44.17)
  line L2 (-11.62, 44.17) -> (-67.5, 44.17)
  line L3 (-120.5, -39.83) -> (67.5, -39.83)
  line L4 (67.5, -39.83) -> (67.5, 39.83)
  circle A2 centre (-58.42, 31.75) radius 3.9
  circle A3 centre (-58.42, -31.75) radius 3.9
  line L5 (-58.42, 31.75) -> (-58.42, -31.75) construction
  line L6 (-58.42, -31.75) -> (58.42, -31.75) construction
  line L7 (58.42, -31.75) -> (58.42, 31.75) construction
  line L8 (58.42, 31.75) -> (-58.42, 31.75) construction
  circle A4 centre (0, 0) radius 1.5
  line L9 (-58.42, 0) -> (58.42, 0) construction
  line L10 (0, -31.75) -> (0, 31.75) construction
  circle A5 centre (-50.8, -24.13) radius 1.5
  circle A6 centre (-38.1, -24.13) radius 1.5
  circle A7 centre (-25.4, -24.13) radius 1.5
  circle A8 centre (-12.7, -24.13) radius 1.5
  circle A9 centre (0, -24.13) radius 1.5
  circle A10 centre (12.7, -24.13) radius 1.5
  circle A11 centre (25.4, -24.13) radius 1.5
  circle A12 centre (38.1, -24.13) radius 1.5
  circle A13 centre (50.8, -24.13) radius 1.5
  circle A14 centre (-50.8, -12.065) radius 1.5
  circle A15 centre (-38.1, -12.065) radius 1.5
  circle A16 centre (-25.4, -12.065) radius 1.5
  circle A17 centre (-12.7, -12.065) radius 1.5
  circle A18 centre (0, -12.065) radius 1.5
  circle A19 centre (12.7, -12.065) radius 1.5
  circle A20 centre (25.4, -12.065) radius 1.5
  circle A21 centre (38.1, -12.065) radius 1.5
  circle A22 centre (50.8, -12.065) radius 1.5
  circle A23 centre (-50.8, 0) radius 1.5
  circle A24 centre (-38.1, 0) radius 1.5
  circle A25 centre (-25.4, 0) radius 1.5
  circle A26 centre (-12.7, 0) radius 1.5
  circle A27 centre (12.7, 0) radius 1.5
  circle A28 centre (25.4, 0) radius 1.5
  circle A29 centre (38.1, 0) radius 1.5
  circle A30 centre (50.8, 0) radius 1.5
  circle A31 centre (-50.8, 12.065) radius 1.5
  circle A32 centre (-38.1, 12.065) radius 1.5
  circle A33 centre (-25.4, 12.065) radius 1.5
  circle A34 centre (-12.7, 12.065) radius 1.5
  circle A35 centre (0, 12.065) radius 1.5
  circle A36 centre (12.7, 12.065) radius 1.5
  circle A37 centre (25.4, 12.065) radius 1.5
  circle A38 centre (38.1, 12.065) radius 1.5
  circle A39 centre (50.8, 12.065) radius 1.5
  circle A40 centre (-50.8, 24.13) radius 1.5
  circle A41 centre (-38.1, 24.13) radius 1.5
  circle A42 centre (-25.4, 24.13) radius 1.5
  circle A43 centre (-12.7, 24.13) radius 1.5
  circle A44 centre (0, 24.13) radius 1.5
  circle A45 centre (12.7, 24.13) radius 1.5
  circle A46 centre (25.4, 24.13) radius 1.5
  circle A47 centre (38.1, 24.13) radius 1.5
  circle A48 centre (50.8, 24.13) radius 1.5
  line L11 (50.8, -24.13) -> (50.8, -12.065) construction
  line L12 (50.8, -12.065) -> (38.1, -12.065) construction
  line L13 (38.1, -12.065) -> (38.1, -24.13) construction
  line L14 (38.1, -24.13) -> (50.8, -24.13) construction
  line L15 (50.8, -18.0975) -> (38.1, -18.0975) construction
  line L16 (44.45, -24.13) -> (44.45, -12.065) construction
  circle A49 centre (44.45, -18.0975) radius 1.5
  circle A50 centre (31.75, -18.0975) radius 1.5
  circle A51 centre (19.05, -18.0975) radius 1.5
  circle A52 centre (6.35, -18.0975) radius 1.5
  circle A53 centre (-6.35, -18.0975) radius 1.5
  circle A54 centre (-19.05, -18.0975) radius 1.5
  circle A55 centre (-31.75, -18.0975) radius 1.5
  circle A56 centre (-44.45, -18.0975) radius 1.5
  circle A57 centre (44.45, -6.0325) radius 1.5
  circle A58 centre (31.75, -6.0325) radius 1.5
  circle A59 centre (19.05, -6.0325) radius 1.5
  circle A60 centre (6.35, -6.0325) radius 1.5
  circle A61 centre (-6.35, -6.0325) radius 1.5
  circle A62 centre (-19.05, -6.0325) radius 1.5
  circle A63 centre (-31.75, -6.0325) radius 1.5
  circle A64 centre (-44.45, -6.0325) radius 1.5
  circle A65 centre (44.45, 6.0325) radius 1.5
  circle A66 centre (31.75, 6.0325) radius 1.5
  circle A67 centre (19.05, 6.0325) radius 1.5
  circle A68 centre (6.35, 6.0325) radius 1.5
  circle A69 centre (-6.35, 6.0325) radius 1.5
  circle A70 centre (-19.05, 6.0325) radius 1.5
  circle A71 centre (-31.75, 6.0325) radius 1.5
  circle A72 centre (-44.45, 6.0325) radius 1.5
  circle A73 centre (44.45, 18.0975) radius 1.5
  circle A74 centre (31.75, 18.0975) radius 1.5
  circle A75 centre (19.05, 18.0975) radius 1.5
  circle A76 centre (6.35, 18.0975) radius 1.5
  circle A77 centre (-6.35, 18.0975) radius 1.5
  circle A78 centre (-19.05, 18.0975) radius 1.5
  circle A79 centre (-31.75, 18.0975) radius 1.5
  circle A80 centre (-44.45, 18.0975) radius 1.5
  line L17 (-115.5, 44.17) -> (-115.5, -27.83)
  line L18 (-115.5, -27.83) -> (-120.5, -27.83)
  line L19 (-120.5, -27.83) -> (-120.5, -39.83)
  line L20 (-67.5, 44.17) -> (-67.5, -22.83)
  line L21 (-67.5, -22.83) -> (-72.5, -22.83)
  line L22 (-72.5, -22.83) -> (-72.5, 44.17)
  line L23 (-72.5, 44.17) -> (-115.5, 44.17)
  dimension "d166" = 50.8
  dimension "d167" = 24.13
  dimension "d168" = 3
  dimension "d171" = 3
  dimension "d174" = -88.9
  dimension "d175" = 36.195
  constraint coincident A2.centre L5.start
  constraint coincident A3.centre L5.end
  constraint coincident A0.centre L6.end
  constraint coincident A1.centre L7.end
  constraint coincident A4.centre origin
  constraint midpoint L5 L9.start
  constraint midpoint L7 L9.end
  constraint midpoint L6 L10.start
  constraint midpoint L8 L10.end
  constraint midpoint L11 L15.start
  constraint midpoint L13 L15.end
  constraint midpoint L14 L16.start
  constraint midpoint L12 L16.end
  constraint midpoint L15 A49.centre
  constraint perpendicular L11 L14
  constraint perpendicular L12 L13
  constraint perpendicular L13 L14
  constraint coincident A22.centre L12
  constraint coincident A22.centre L11
  constraint coincident A12.centre L13
  constraint coincident A12.centre L14
  constraint coincident A13.centre L11.start
  measures "d168" diameter of A4
  measures "d171" diameter of A49
extrude "Extrude21" cut sketch "Sketch17" against normal up to surface (5 mm away) contours A4 | A5 | A6 | A7 | A8 | A9 | A10 | A11 | A12 | A13 | A14 | A15 | A16 | A17 | A18 | A19 | A20 | A21 | A22 | A23 | A24 | A25 | A26 | A27 | A28 | A29 | A30 | A31 | A32 | A33 | A34 | A35 | A36 | A37 | A38 | A39 | A40 | A41 | A42 | A43 | A44 | A45 | A46 | A47 | A48 | A49 | A50 | A51 | A52 | A53 | A54 | A55 | A56 | A57 | A58 | A59 | A60 | A61 | A62 | A63 | A64 | A65 | A66 | A67 | A68 | A69 | A70 | A71 | A72 | A73 | A74 | A75 | A76 | A77 | A78 | A79 | A80 bodies 1
sketch "Sketch18" plane through (0, 5, 0) normal (0, 1, 0) x (-1, 0, 0)
  line L0 (-11.62, 44.17) -> (-67.5, 44.17)
  line L1 (-115.5, 44.17) -> (-115.5, -27.83)
  line L2 (-115.5, -27.83) -> (-120.5, -27.83)
  line L3 (-120.5, -27.83) -> (-120.5, -39.83)
  line L4 (-120.5, -39.83) -> (67.5, -39.83)
  circle A0 centre (-31.75, 6.0325) radius 1.5
  circle A1 centre (-31.75, -18.0975) radius 1.5
  circle A2 centre (-6.35, -18.0975) radius 1.5
  circle A3 centre (-6.35, 18.0975) radius 1.5
  circle A4 centre (19.05, 18.0975) radius 1.5
  circle A5 centre (6.35, -18.0975) radius 1.5
  circle A6 centre (31.75, 6.0325) radius 1.5
  circle A7 centre (44.45, -6.0325) radius 1.5
  circle A8 centre (38.1, 24.13) radius 1.5
  circle A9 centre (0, 24.13) radius 1.5
  circle A10 centre (-25.4, -24.13) radius 1.5
  circle A11 centre (-12.7, -24.13) radius 1.5
  circle A12 centre (12.7, 12.065) radius 1.5
  circle A13 centre (50.8, -24.13) radius 1.5
  circle A14 centre (-50.8, -24.13) radius 1.5
  circle A15 centre (12.7, -12.065) radius 1.5
  circle A16 centre (-25.4, -12.065) radius 1.5
  circle A17 centre (50.8, 12.065) radius 1.5
  circle A18 centre (-38.1, 0) radius 1.5
  circle A19 centre (-50.8, 24.13) radius 1.5
  circle A20 centre (-12.7, -12.065) radius 1.5
  circle A21 centre (-38.1, -12.065) radius 1.5
  circle A22 centre (-38.1, -24.13) radius 1.5
  circle A23 centre (25.4, 0) radius 1.5
  circle A24 centre (25.4, -24.13) radius 1.5
  circle A25 centre (12.7, -24.13) radius 1.5
  circle A26 centre (38.1, -12.065) radius 1.5
  circle A27 centre (-38.1, 24.13) radius 1.5
  circle A28 centre (0, 12.065) radius 1.5
  circle A29 centre (-25.4, 0) radius 1.5
  circle A30 centre (44.45, -18.0975) radius 1.5
  circle A31 centre (31.75, 18.0975) radius 1.5
  circle A32 centre (19.05, -18.0975) radius 1.5
  circle A33 centre (19.05, 6.0325) radius 1.5
  circle A34 centre (-6.35, 6.0325) radius 1.5
  circle A35 centre (-6.35, -6.0325) radius 1.5
  circle A36 centre (-31.75, -6.0325) radius 1.5
  circle A37 centre (-44.45, 6.0325) radius 1.5
  circle A38 centre (-31.75, 18.0975) radius 1.5
  circle A39 centre (-44.45, -18.0975) radius 1.5
  circle A40 centre (-19.05, -18.0975) radius 1.5
  circle A41 centre (-19.05, 18.0975) radius 1.5
  circle A42 centre (6.35, 18.0975) radius 1.5
  circle A43 centre (6.35, -6.0325) radius 1.5
  circle A44 centre (31.75, -6.0325) radius 1.5
  circle A45 centre (44.45, 6.0325) radius 1.5
  circle A46 centre (25.4, 24.13) radius 1.5
  circle A47 centre (38.1, 0) radius 1.5
  circle A48 centre (-50.8, -12.065) radius 1.5
  circle A49 centre (-25.4, 24.13) radius 1.5
  circle A50 centre (-38.1, 12.065) radius 1.5
  circle A51 centre (38.1, -24.13) radius 1.5
  circle A52 centre (-50.8, 0) radius 1.5
  circle A53 centre (50.8, -12.065) radius 1.5
  circle A54 centre (38.1, 12.065) radius 1.5
  circle A55 centre (-50.8, 12.065) radius 1.5
  circle A56 centre (0, -24.13) radius 1.5
  circle A57 centre (-12.7, 0) radius 1.5
  circle A58 centre (12.7, 24.13) radius 1.5
  circle A59 centre (25.4, 12.065) radius 1.5
  circle A60 centre (-25.4, 12.065) radius 1.5
  circle A61 centre (12.7, 0) radius 1.5
  circle A62 centre (-12.7, 24.13) radius 1.5
  circle A63 centre (25.4, -12.065) radius 1.5
  circle A64 centre (0, 0) radius 1.5
  circle A65 centre (50.8, 0) radius 1.5
  circle A66 centre (50.8, 24.13) radius 1.5
  circle A67 centre (0, -12.065) radius 1.5
  circle A68 centre (-12.7, 12.065) radius 1.5
  circle A69 centre (44.45, 18.0975) radius 1.5
  circle A70 centre (31.75, -18.0975) radius 1.5
  circle A71 centre (19.05, -6.0325) radius 1.5
  circle A72 centre (6.35, 6.0325) radius 1.5
  circle A73 centre (-19.05, 6.0325) radius 1.5
  circle A74 centre (-19.05, -6.0325) radius 1.5
  circle A75 centre (-44.45, -6.0325) radius 1.5
  circle A76 centre (-44.45, 18.0975) radius 1.5
  circle A77 centre (58.42, -31.75) radius 3.9
  circle A78 centre (58.42, 31.75) radius 3.9
  line L5 (67.5, 39.83) -> (-11.62, 39.83)
  line L6 (-11.62, 39.83) -> (-11.62, 44.17)
  line L7 (67.5, -39.83) -> (67.5, 39.83)
  circle A79 centre (-58.42, 31.75) radius 3.9
  circle A80 centre (-58.42, -31.75) radius 3.9
  line L8 (-67.5, 44.17) -> (-67.5, -22.83)
  line L9 (-67.5, -22.83) -> (-72.5, -22.83)
  line L10 (-72.5, -22.83) -> (-72.5, 44.17)
  line L11 (-72.5, 44.17) -> (-115.5, 44.17)